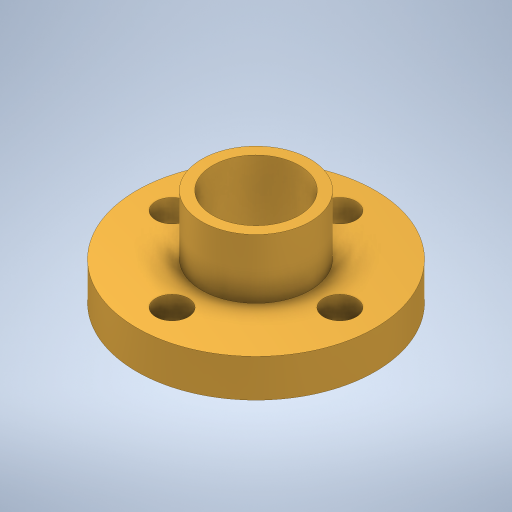
# Autodesk Inventor part: ACME Brass Nut
Saved by Autodesk Inventor 2023.1 (Build 271208000, 208)
## iProperties
Created: 2023-01-19
Part Number: ACME Brass Nut
Material: Brass, Soft Yellow
Document SubType Name: Modeling
Designer: dmargari
Density: 8.47 g/cm^3
Appearance: Brass - Satin
Author: dmargari
Autodesk Inventor part; units mm, degrees
ref_plane "YZ Plane" through (0, 0, 0) normal (1, 0, 0) x (0, 1, 0)
ref_plane "XZ Plane" through (0, 0, 0) normal (0, 1, 0) x (-1, 0, 0)
ref_plane "XY Plane" through (0, 0, 0) normal (0, 0, 1) x (1, 0, 0)
sketch "Sketch1" plane through (0, 0, 0) normal (0, 1, 0) x (-1, 0, 0)
  circle A0 centre (22.2894, -21.943) radius 11
  circle A1 centre (22.2894, -21.943) radius 7.75 construction
  circle A2 centre (22.2894, -21.943) radius 5
  circle A3 centre (22.2894, -21.943) radius 4
  point P0 (0, 0)
  point P1 (14.5394, -21.943)
  dimension "d2" = 15.5
  dimension "d1" = 22
  dimension "d4" = 10
  dimension "d17" = 8
  constraints: 3 centre point, 3 coincident, 1 horizontal alignment, 2 other
  measures "d1" diameter of A0
  measures "d4" diameter of A2
  measures "d17" diameter of A3
extrude "Extrusion1" add sketch "Sketch1" along normal blind 3.5 contours A0
hole "Hole1" at (-14.5394, 0, -21.943) direction (0, 1, 0) diameter 3 end through all countersink diameter 4 countersink angle 90
pattern_circular "Circular Pattern1" count 4 over 360 about axis through (-22.2894, 0, -21.943) along (0, 1, 0) of "Hole1"
extrude "Extrusion2" add sketch "Sketch1" along normal blind 9 and the other way blind 1.5 contours A2
